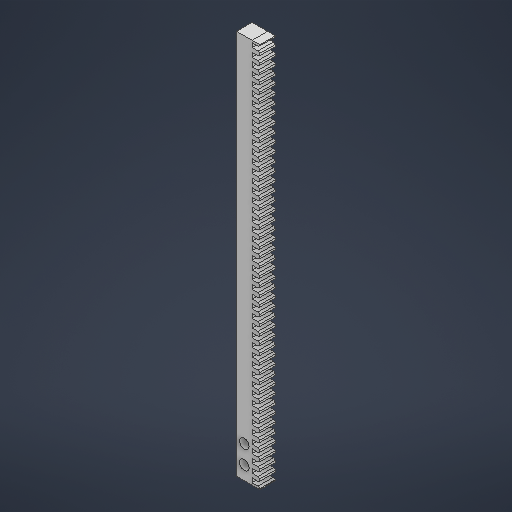
# Autodesk Inventor part: Gear-Rack
Saved by Autodesk Inventor 2026.2 (Build 302298010, 298A)
## iProperties
Created: 2026-05-26
Part Number: Gear-Rack
Material: Genérico
Document SubType Name: Modeling
Designer: pauli
Density: 1 g/cm^3
Appearance: Padrão
Author: pauli
Autodesk Inventor part; units mm, degrees
ref_plane "YZ Plane" through (0, 0, 0) normal (1, 0, 0) x (0, 1, 0)
ref_plane "XZ Plane" through (0, 0, 0) normal (0, 1, 0) x (-1, 0, 0)
ref_plane "XY Plane" through (0, 0, 0) normal (0, 0, 1) x (1, 0, 0)
sketch "Esboço1" plane through (0, 0, 0) normal (0, 0, 1) x (1, 0, 0)
  line L0 (2, 49.518) -> (-2, 49.518)
  line L1 (-2, 49.518) -> (-2, -49.518)
  line L2 (-2, -49.518) -> (2, -49.518)
  line L3 (2, -49.518) -> (2, 49.518)
  line L4 (2, 49.518) -> (-2, -49.518) construction
  line L5 (-2, 49.518) -> (2, -49.518) construction
  line L6 (2, -49.518) -> (4, -49.518)
  line L7 (2, -49.518) -> (4, -49.518) construction
  line L8 (4, -49.518) -> (4, -49.268)
  line L9 (4, -49.268) -> (3.5, -48.9793)
  line L10 (3.5, -48.9793) -> (2, -48.9793)
  line L11 (2, -48.9793) -> (2, -48.4413) construction
  line L12 (2, -48.4413) -> (4.1439, -48.4413) construction
  line L13 (2, -47.3646) -> (4, -47.3646) construction
  line L14 (2, -47.3646) -> (4, -47.3646) construction
  line L15 (4, -47.3646) -> (4, -47.6146)
  line L16 (4, -47.6146) -> (3.5, -47.9033)
  line L17 (3.5, -47.9033) -> (2, -47.9033)
  line L18 (3.5, -45.7503) -> (2, -45.7503)
  line L19 (4, -45.4616) -> (3.5, -45.7503)
  line L20 (4, -45.2116) -> (4, -45.4616)
  line L21 (3.5, -46.8263) -> (2, -46.8263)
  line L22 (4, -47.115) -> (3.5, -46.8263)
  line L23 (4, -47.365) -> (4, -47.115)
  line L24 (3.5, -43.5973) -> (2, -43.5973)
  line L25 (4, -43.3086) -> (3.5, -43.5973)
  line L26 (4, -43.0586) -> (4, -43.3086)
  line L27 (3.5, -44.6733) -> (2, -44.6733)
  line L28 (4, -44.962) -> (3.5, -44.6733)
  line L29 (4, -45.212) -> (4, -44.962)
  line L30 (3.5, -41.4443) -> (2, -41.4443)
  line L31 (4, -41.1556) -> (3.5, -41.4443)
  line L32 (4, -40.9056) -> (4, -41.1556)
  line L33 (3.5, -42.5203) -> (2, -42.5203)
  line L34 (4, -42.809) -> (3.5, -42.5203)
  line L35 (4, -43.059) -> (4, -42.809)
  line L36 (3.5, -39.2913) -> (2, -39.2913)
  line L37 (4, -39.0026) -> (3.5, -39.2913)
  line L38 (4, -38.7526) -> (4, -39.0026)
  line L39 (3.5, -40.3673) -> (2, -40.3673)
  line L40 (4, -40.656) -> (3.5, -40.3673)
  line L41 (4, -40.906) -> (4, -40.656)
  line L42 (3.5, -37.1383) -> (2, -37.1383)
  line L43 (4, -36.8496) -> (3.5, -37.1383)
  line L44 (4, -36.5996) -> (4, -36.8496)
  line L45 (3.5, -38.2143) -> (2, -38.2143)
  line L46 (4, -38.503) -> (3.5, -38.2143)
  line L47 (4, -38.753) -> (4, -38.503)
  line L48 (3.5, -34.9853) -> (2, -34.9853)
  line L49 (4, -34.6966) -> (3.5, -34.9853)
  line L50 (4, -34.4466) -> (4, -34.6966)
  line L51 (3.5, -36.0613) -> (2, -36.0613)
  line L52 (4, -36.35) -> (3.5, -36.0613)
  line L53 (4, -36.6) -> (4, -36.35)
  line L54 (3.5, -32.8323) -> (2, -32.8323)
  line L55 (4, -32.5436) -> (3.5, -32.8323)
  line L56 (4, -32.2936) -> (4, -32.5436)
  line L57 (3.5, -33.9083) -> (2, -33.9083)
  line L58 (4, -34.197) -> (3.5, -33.9083)
  line L59 (4, -34.447) -> (4, -34.197)
  line L60 (3.5, -30.6793) -> (2, -30.6793)
  line L61 (4, -30.3906) -> (3.5, -30.6793)
  line L62 (4, -30.1406) -> (4, -30.3906)
  line L63 (3.5, -31.7553) -> (2, -31.7553)
  line L64 (4, -32.044) -> (3.5, -31.7553)
  line L65 (4, -32.294) -> (4, -32.044)
  line L66 (3.5, -28.5263) -> (2, -28.5263)
  line L67 (4, -28.2376) -> (3.5, -28.5263)
  line L68 (4, -27.9876) -> (4, -28.2376)
  line L69 (3.5, -29.6023) -> (2, -29.6023)
  line L70 (4, -29.891) -> (3.5, -29.6023)
  line L71 (4, -30.141) -> (4, -29.891)
  line L72 (3.5, -26.3733) -> (2, -26.3733)
  line L73 (4, -26.0846) -> (3.5, -26.3733)
  line L74 (4, -25.8346) -> (4, -26.0846)
  line L75 (3.5, -27.4493) -> (2, -27.4493)
  line L76 (4, -27.738) -> (3.5, -27.4493)
  line L77 (4, -27.988) -> (4, -27.738)
  line L78 (3.5, -24.2203) -> (2, -24.2203)
  line L79 (4, -23.9316) -> (3.5, -24.2203)
  line L80 (4, -23.6816) -> (4, -23.9316)
  line L81 (3.5, -25.2963) -> (2, -25.2963)
  line L82 (4, -25.585) -> (3.5, -25.2963)
  line L83 (4, -25.835) -> (4, -25.585)
  line L84 (3.5, -22.0673) -> (2, -22.0673)
  line L85 (4, -21.7786) -> (3.5, -22.0673)
  line L86 (4, -21.5286) -> (4, -21.7786)
  line L87 (3.5, -23.1433) -> (2, -23.1433)
  line L88 (4, -23.432) -> (3.5, -23.1433)
  line L89 (4, -23.682) -> (4, -23.432)
  line L90 (3.5, -19.9143) -> (2, -19.9143)
  line L91 (4, -19.6256) -> (3.5, -19.9143)
  line L92 (4, -19.3756) -> (4, -19.6256)
  line L93 (3.5, -20.9903) -> (2, -20.9903)
  line L94 (4, -21.279) -> (3.5, -20.9903)
  line L95 (4, -21.529) -> (4, -21.279)
  line L96 (3.5, -17.7613) -> (2, -17.7613)
  line L97 (4, -17.4726) -> (3.5, -17.7613)
  line L98 (4, -17.2226) -> (4, -17.4726)
  line L99 (3.5, -18.8373) -> (2, -18.8373)
  line L100 (4, -19.126) -> (3.5, -18.8373)
  line L101 (4, -19.376) -> (4, -19.126)
  line L102 (3.5, -15.6083) -> (2, -15.6083)
  line L103 (4, -15.3196) -> (3.5, -15.6083)
  line L104 (4, -15.0696) -> (4, -15.3196)
  line L105 (3.5, -16.6843) -> (2, -16.6843)
  line L106 (4, -16.973) -> (3.5, -16.6843)
  line L107 (4, -17.223) -> (4, -16.973)
  line L108 (3.5, -13.4553) -> (2, -13.4553)
  line L109 (4, -13.1666) -> (3.5, -13.4553)
  line L110 (4, -12.9166) -> (4, -13.1666)
  line L111 (3.5, -14.5313) -> (2, -14.5313)
  line L112 (4, -14.82) -> (3.5, -14.5313)
  line L113 (4, -15.07) -> (4, -14.82)
  line L114 (3.5, -11.3023) -> (2, -11.3023)
  line L115 (4, -11.0136) -> (3.5, -11.3023)
  line L116 (4, -10.7636) -> (4, -11.0136)
  line L117 (3.5, -12.3783) -> (2, -12.3783)
  line L118 (4, -12.667) -> (3.5, -12.3783)
  line L119 (4, -12.917) -> (4, -12.667)
  line L120 (3.5, -9.1493) -> (2, -9.1493)
  line L121 (4, -8.8606) -> (3.5, -9.1493)
  line L122 (4, -8.6106) -> (4, -8.8606)
  line L123 (3.5, -10.2253) -> (2, -10.2253)
  line L124 (4, -10.514) -> (3.5, -10.2253)
  line L125 (4, -10.764) -> (4, -10.514)
  line L126 (3.5, -6.9963) -> (2, -6.9963)
  line L127 (4, -6.7076) -> (3.5, -6.9963)
  line L128 (4, -6.4576) -> (4, -6.7076)
  line L129 (3.5, -8.0723) -> (2, -8.0723)
  line L130 (4, -8.361) -> (3.5, -8.0723)
  line L131 (4, -8.611) -> (4, -8.361)
  line L132 (3.5, -4.8433) -> (2, -4.8433)
  line L133 (4, -4.5546) -> (3.5, -4.8433)
  line L134 (4, -4.3046) -> (4, -4.5546)
  line L135 (3.5, -5.9193) -> (2, -5.9193)
  line L136 (4, -6.208) -> (3.5, -5.9193)
  line L137 (4, -6.458) -> (4, -6.208)
  line L138 (3.5, -2.6903) -> (2, -2.6903)
  line L139 (4, -2.4016) -> (3.5, -2.6903)
  line L140 (4, -2.1516) -> (4, -2.4016)
  line L141 (3.5, -3.7663) -> (2, -3.7663)
  line L142 (4, -4.055) -> (3.5, -3.7663)
  line L143 (4, -4.305) -> (4, -4.055)
  line L144 (3.5, -0.5373) -> (2, -0.5373)
  line L145 (4, -0.2486) -> (3.5, -0.5373)
  line L146 (4, 0.0014) -> (4, -0.2486)
  line L147 (3.5, -1.6133) -> (2, -1.6133)
  line L148 (4, -1.902) -> (3.5, -1.6133)
  line L149 (4, -2.152) -> (4, -1.902)
  line L150 (3.5, 1.6157) -> (2, 1.6157)
  line L151 (4, 1.9044) -> (3.5, 1.6157)
  line L152 (4, 2.1544) -> (4, 1.9044)
  line L153 (3.5, 0.5397) -> (2, 0.5397)
  line L154 (4, 0.251) -> (3.5, 0.5397)
  line L155 (4, 0.001) -> (4, 0.251)
  line L156 (3.5, 3.7687) -> (2, 3.7687)
  line L157 (4, 4.0574) -> (3.5, 3.7687)
  line L158 (4, 4.3074) -> (4, 4.0574)
  line L159 (3.5, 2.6927) -> (2, 2.6927)
  line L160 (4, 2.404) -> (3.5, 2.6927)
  line L161 (4, 2.154) -> (4, 2.404)
  line L162 (3.5, 5.9217) -> (2, 5.9217)
  line L163 (4, 6.2104) -> (3.5, 5.9217)
  line L164 (4, 6.4604) -> (4, 6.2104)
  line L165 (3.5, 4.8457) -> (2, 4.8457)
  line L166 (4, 4.557) -> (3.5, 4.8457)
  line L167 (4, 4.307) -> (4, 4.557)
  line L168 (3.5, 8.0747) -> (2, 8.0747)
  line L169 (4, 8.3634) -> (3.5, 8.0747)
  line L170 (4, 8.6134) -> (4, 8.3634)
  line L171 (3.5, 6.9987) -> (2, 6.9987)
  line L172 (4, 6.71) -> (3.5, 6.9987)
  line L173 (4, 6.46) -> (4, 6.71)
  line L174 (3.5, 10.2277) -> (2, 10.2277)
  line L175 (4, 10.5164) -> (3.5, 10.2277)
  line L176 (4, 10.7664) -> (4, 10.5164)
  line L177 (3.5, 9.1517) -> (2, 9.1517)
  line L178 (4, 8.863) -> (3.5, 9.1517)
  line L179 (4, 8.613) -> (4, 8.863)
  line L180 (3.5, 12.3807) -> (2, 12.3807)
  line L181 (4, 12.6694) -> (3.5, 12.3807)
  line L182 (4, 12.9194) -> (4, 12.6694)
  line L183 (3.5, 11.3047) -> (2, 11.3047)
  line L184 (4, 11.016) -> (3.5, 11.3047)
  line L185 (4, 10.766) -> (4, 11.016)
  line L186 (3.5, 14.5337) -> (2, 14.5337)
  line L187 (4, 14.8224) -> (3.5, 14.5337)
  line L188 (4, 15.0724) -> (4, 14.8224)
  line L189 (3.5, 13.4577) -> (2, 13.4577)
  line L190 (4, 13.169) -> (3.5, 13.4577)
  line L191 (4, 12.919) -> (4, 13.169)
  line L192 (3.5, 16.6867) -> (2, 16.6867)
  line L193 (4, 16.9754) -> (3.5, 16.6867)
  line L194 (4, 17.2254) -> (4, 16.9754)
  line L195 (3.5, 15.6107) -> (2, 15.6107)
  line L196 (4, 15.322) -> (3.5, 15.6107)
  line L197 (4, 15.072) -> (4, 15.322)
  line L198 (3.5, 18.8397) -> (2, 18.8397)
  line L199 (4, 19.1284) -> (3.5, 18.8397)
  line L200 (4, 19.3784) -> (4, 19.1284)
  line L201 (3.5, 17.7637) -> (2, 17.7637)
  line L202 (4, 17.475) -> (3.5, 17.7637)
  line L203 (4, 17.225) -> (4, 17.475)
  line L204 (3.5, 20.9927) -> (2, 20.9927)
  line L205 (4, 21.2814) -> (3.5, 20.9927)
  line L206 (4, 21.5314) -> (4, 21.2814)
  line L207 (3.5, 19.9167) -> (2, 19.9167)
  line L208 (4, 19.628) -> (3.5, 19.9167)
  line L209 (4, 19.378) -> (4, 19.628)
  line L210 (3.5, 23.1457) -> (2, 23.1457)
  line L211 (4, 23.4344) -> (3.5, 23.1457)
  line L212 (4, 23.6844) -> (4, 23.4344)
  line L213 (3.5, 22.0697) -> (2, 22.0697)
  line L214 (4, 21.781) -> (3.5, 22.0697)
  line L215 (4, 21.531) -> (4, 21.781)
  line L216 (3.5, 25.2987) -> (2, 25.2987)
  line L217 (4, 25.5874) -> (3.5, 25.2987)
  line L218 (4, 25.8374) -> (4, 25.5874)
  line L219 (3.5, 24.2227) -> (2, 24.2227)
  line L220 (4, 23.934) -> (3.5, 24.2227)
  line L221 (4, 23.684) -> (4, 23.934)
  line L222 (3.5, 27.4517) -> (2, 27.4517)
  line L223 (4, 27.7404) -> (3.5, 27.4517)
  line L224 (4, 27.9904) -> (4, 27.7404)
  line L225 (3.5, 26.3757) -> (2, 26.3757)
  line L226 (4, 26.087) -> (3.5, 26.3757)
  line L227 (4, 25.837) -> (4, 26.087)
  line L228 (3.5, 29.6047) -> (2, 29.6047)
  line L229 (4, 29.8934) -> (3.5, 29.6047)
  line L230 (4, 30.1434) -> (4, 29.8934)
  line L231 (3.5, 28.5287) -> (2, 28.5287)
  line L232 (4, 28.24) -> (3.5, 28.5287)
  line L233 (4, 27.99) -> (4, 28.24)
  line L234 (3.5, 31.7577) -> (2, 31.7577)
  line L235 (4, 32.0464) -> (3.5, 31.7577)
  line L236 (4, 32.2964) -> (4, 32.0464)
  line L237 (3.5, 30.6817) -> (2, 30.6817)
  line L238 (4, 30.393) -> (3.5, 30.6817)
  line L239 (4, 30.143) -> (4, 30.393)
  line L240 (3.5, 33.9107) -> (2, 33.9107)
  line L241 (4, 34.1994) -> (3.5, 33.9107)
  line L242 (4, 34.4494) -> (4, 34.1994)
  line L243 (3.5, 32.8347) -> (2, 32.8347)
  line L244 (4, 32.546) -> (3.5, 32.8347)
  line L245 (4, 32.296) -> (4, 32.546)
  line L246 (3.5, 36.0637) -> (2, 36.0637)
  line L247 (4, 36.3524) -> (3.5, 36.0637)
  line L248 (4, 36.6024) -> (4, 36.3524)
  line L249 (3.5, 34.9877) -> (2, 34.9877)
  line L250 (4, 34.699) -> (3.5, 34.9877)
  line L251 (4, 34.449) -> (4, 34.699)
  line L252 (3.5, 38.2167) -> (2, 38.2167)
  line L253 (4, 38.5054) -> (3.5, 38.2167)
  line L254 (4, 38.7554) -> (4, 38.5054)
  line L255 (3.5, 37.1407) -> (2, 37.1407)
  line L256 (4, 36.852) -> (3.5, 37.1407)
  line L257 (4, 36.602) -> (4, 36.852)
  line L258 (3.5, 40.3697) -> (2, 40.3697)
  line L259 (4, 40.6584) -> (3.5, 40.3697)
  line L260 (4, 40.9084) -> (4, 40.6584)
  line L261 (3.5, 39.2937) -> (2, 39.2937)
  line L262 (4, 39.005) -> (3.5, 39.2937)
  line L263 (4, 38.755) -> (4, 39.005)
  line L264 (3.5, 42.5227) -> (2, 42.5227)
  line L265 (4, 42.8114) -> (3.5, 42.5227)
  line L266 (4, 43.0614) -> (4, 42.8114)
  line L267 (3.5, 41.4467) -> (2, 41.4467)
  line L268 (4, 41.158) -> (3.5, 41.4467)
  line L269 (4, 40.908) -> (4, 41.158)
  line L270 (3.5, 44.6757) -> (2, 44.6757)
  line L271 (4, 44.9644) -> (3.5, 44.6757)
  line L272 (4, 45.2144) -> (4, 44.9644)
  line L273 (3.5, 43.5997) -> (2, 43.5997)
  line L274 (4, 43.311) -> (3.5, 43.5997)
  line L275 (4, 43.061) -> (4, 43.311)
  line L276 (3.5, 46.8287) -> (2, 46.8287)
  line L277 (4, 47.1174) -> (3.5, 46.8287)
  line L278 (4, 47.3674) -> (4, 47.1174)
  line L279 (3.5, 45.7527) -> (2, 45.7527)
  line L280 (4, 45.464) -> (3.5, 45.7527)
  line L281 (4, 45.214) -> (4, 45.464)
  line L282 (3.5, 48.9817) -> (2, 48.9817)
  line L283 (4, 49.2704) -> (3.5, 48.9817)
  line L284 (4, 49.5204) -> (4, 49.2704)
  line L285 (3.5, 47.9057) -> (2, 47.9057)
  line L286 (4, 47.617) -> (3.5, 47.9057)
  line L287 (4, 47.367) -> (4, 47.617)
  line L288 (2, 49.518) -> (4, 49.5204)
  point P0 (0, 0)
  dimension "d0" = 4
  dimension "d1" = 99.036
  dimension "d2" = 2
  dimension "d3" = 0
  dimension "d4" = 0.25
  dimension "d5" = 120
  dimension "d6" = 0.5
  dimension "d7" = 0.538
  dimension "d10" = 2.153
  constraints: 576 end point, 360 vertical alignment, 181 parallel, 91 collinear, 6 symmetric about line, 4 horizontal, 2 midpoint, 2 perpendicular, 2 vertical, 4 other
  measures "d0" distance of L2.end L1.end
  measures "d1" distance of L1.end L0.end
  measures "d2" distance of L2.end L6.end
  measures "d3" distance between parallel lines of L6 L7
  measures "d4" distance of L7.end L8.end
  measures "d5" angle of L9 L8
  measures "d6" horizontal distance of L8.end L9.end
  measures "d7" distance of L10.end L11.end
  measures "d10" distance of L17.start L18.start
extrude "Extrusão1" add sketch "Esboço1" along normal blind 4
sketch "Esboço2" plane through (0, 0, 4) normal (0, 0, 1) x (1, 0, 0)
  line L0 (-2, 49.518) -> (-2, -49.518) projected
  line L1 (-2, 0) -> (-2, -49.518)
  line L2 (-2, -49.518) -> (4, -49.518) projected
  line L3 (-2, -49.518) -> (0, -49.518)
  line L4 (0, -49.518) -> (0, -47.518)
  line L5 (0, -47.518) -> (0, -46.018)
  circle A0 centre (0, -46.018) radius 1.25
  line L6 (0, -46.018) -> (0, -44.768)
  line L7 (0, -44.768) -> (0, -41.268)
  circle A1 centre (0, -41.268) radius 1.25
  point P0 (0, 0)
  dimension "d19" = 2.5
  dimension "d17" = 2
  dimension "d18" = 1.5
  dimension "d20" = 3.5
  dimension "d21" = 2.5
  constraints: 12 end point, 3 vertical, 2 coincident, 2 point on line, 1 centre point, 1 collinear, 1 midpoint, 1 vertical alignment, 2 other
  measures "d17" distance of L3.end L4.end
  measures "d18" distance of L4.end L5.end
  measures "d20" distance of L6.end L7.end
  measures "d21" diameter of A1
extrude "Extrusão2" cut sketch "Esboço2" against normal blind 4
